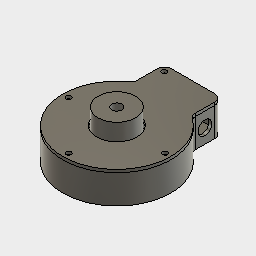
hihatController (Autodesk Fusion 360 design; units mm, degrees)
Autodesk Fusion 360 part; units mm, degrees
sketch "スケッチ1" plane through (0, 0, 0) normal (0, 1, 0) x (1, 0, 0)
  line L0 (-22, 22) -> (22, 22)
  line L1 (22, 22) -> (22, -22)
  line L2 (22, -22) -> (-22, -22)
  line L3 (-22, -22) -> (-22, 22)
  circle A0 centre (0, 0) radius 6.5
  circle A1 centre (0, 0) radius 37.5
  circle A2 centre (0, 0) radius 34.5
  line L4 (0, 47) -> (17.5, 47)
  line L5 (0, 47) -> (-17.5, 47)
  line L6 (-17.5, 47) -> (-17.5, 33.1662)
  line L7 (17.5, 47) -> (17.5, 33.1662)
  line L8 (-20.5, 33.1662) -> (-20.5, 31.4006)
  line L9 (20.5, 33.1662) -> (20.5, 31.4006)
  line L10 (-20.5, 31.4006) -> (-20.5, 25)
  line L11 (-17.5, 33.1662) -> (-17.5, 27)
  line L12 (17.5, 33.1662) -> (17.5, 26)
  line L13 (20.5, 31.4006) -> (20.5, 26)
  line L14 (-20.5, 50) -> (-20.5, 33.1662)
  line L15 (0, 50) -> (-20.5, 50)
  line L16 (0, 50) -> (20.5, 50)
  line L17 (20.5, 50) -> (20.5, 33.1662)
  dimension "d18" = 3
extrude "押し出し1" add sketch "スケッチ1" along normal blind 40 contours A1 A2 L10 L13 | A1 A2 L12 L13 | A1 L4 L5 L6 L7 L8 L9 L14 L15 L16 L17 | A1 A2 L10 L11 makes body 1
extrude "押し出し2" add sketch "スケッチ1" along normal blind 3 contours L0 L1 L2 L3 | A1 A2 L11 L12 | A1 L4 L5 L6 L7 | A2 bodies 1
fillet "フィレット1" radius 10 2 edges at (20.5, 20, -31.4006) (-20.5, 20, -31.4006) on bodies 1
fillet "フィレット2" radius 5 2 edges at (-20.5, 20, -50) (20.5, 20, -50) on bodies 1
fillet "フィレット3" radius 2 2 edges at (-17.5, 21.5, -47) (17.5, 21.5, -47) on bodies 1
sketch "スケッチ2" plane through (20.5, 0, 0) normal (1, 0, 0) x (0, 0, -1)
  line L0 (45, 0) -> (45, 40)
  line L1 (45, 40) -> (36.4143, 40)
  line L2 (36.4143, 40) -> (36.4143, 0)
  line L3 (36.4143, 0) -> (45, 0)
  line L4 (40.7071, 0) -> (40.7071, 10)
  circle A0 centre (40.7071, 10) radius 4.75
  dimension "d26" = 10
  dimension "d27" = 9.5
  measures "d26" distance of L4.start L4.end
  measures "d27" diameter of A0
extrude "押し出し3" cut sketch "スケッチ2" along normal mid plane 14 contours L0 L2 A0 | L0 A0 | L2 A0 bodies 1
sketch "スケッチ3" plane through (0, 40, 0) normal (0, 1, 0) x (-1, 0, 0)
  arc A0 (-20.5, -45) -> (-15.5, -50) centre (-15.5, -45) ccw
  line L0 (-15.5, -50) -> (15.5, -50)
  arc A1 (15.5, -50) -> (20.5, -45) centre (15.5, -45) ccw
  line L1 (20.5, -45) -> (20.5, -36.4143)
  arc A2 (24.0789, -28.7481) -> (20.5, -36.4143) centre (30.5, -36.4143) ccw
  arc A3 (24.0789, -28.7481) -> (-24.0789, -28.7481) centre (0, 0) ccw
  arc A4 (-20.5, -36.4143) -> (-24.0789, -28.7481) centre (-30.5, -36.4143) ccw
  line L2 (-20.5, -36.4143) -> (-20.5, -45)
  line L3 (15.5, -47) -> (-15.5, -47)
  arc A5 (-17.5, -45) -> (-15.5, -47) centre (-15.5, -45) ccw
  line L4 (-17.5, -45) -> (-17.5, -29.7321)
  arc A6 (17.5, -29.7321) -> (-17.5, -29.7321) centre (0, 0) ccw
  line L5 (17.5, -29.7321) -> (17.5, -45)
  arc A7 (15.5, -47) -> (17.5, -45) centre (15.5, -45) ccw
  circle A8 centre (0, 0) radius 37.5
  circle A9 centre (0, 0) radius 37.5
  circle A10 centre (0, 0) radius 34.5
  circle A11 centre (0, 0) radius 34.5
  circle A12 centre (0, 0) radius 56.7387
  point P0 (-10.5, -40)
  point P1 (10.5, -40)
extrude "押し出し4" cut sketch "スケッチ3" against normal blind 20 contours A0 L0 A1 L1 A2 A4 L2 L3 A5 L4 L5 A7 A8 A9 | L3 A5 L4 L5 A7 A8 A9 | A12 bodies 1
extrude "押し出し5" add sketch "スケッチ3" against normal blind 20 contours L4 L5 A8 A9 A10 A11 bodies 1
sketch "スケッチ4" plane through (0, 20, 0) normal (0, 1, 0) x (-1, 0, 0)
  line L0 (17.5, -33.1662) -> (17.5, -45)
  arc A0 (15.5, -47) -> (17.5, -45) centre (15.5, -45) ccw
  line L1 (15.5, -47) -> (-15.5, -47)
  arc A1 (-17.5, -45) -> (-15.5, -47) centre (-15.5, -45) ccw
  line L2 (-17.5, -45) -> (-17.5, -33.1662)
  arc A2 (-24.0789, -28.7481) -> (-17.5, -33.1662) centre (0, 0) ccw
  arc A3 (-20.5, -36.4143) -> (-24.0789, -28.7481) centre (-30.5, -36.4143) ccw
  line L3 (-20.5, -36.4143) -> (-20.5, -45)
  arc A4 (-20.5, -45) -> (-15.5, -50) centre (-15.5, -45) ccw
  line L4 (-15.5, -50) -> (15.5, -50)
  arc A5 (15.5, -50) -> (20.5, -45) centre (15.5, -45) ccw
  line L5 (20.5, -45) -> (20.5, -36.4143)
  arc A6 (24.0789, -28.7481) -> (20.5, -36.4143) centre (30.5, -36.4143) ccw
  arc A7 (17.5, -33.1662) -> (24.0789, -28.7481) centre (0, 0) ccw
  circle A8 centre (0, 0) radius 37.5
  arc A9 (-17.5, -33.1662) -> (17.5, -33.1662) centre (0, 0) ccw
  circle A10 centre (0, 0) radius 37.5
  point P0 (-15.5, -45)
  point P1 (15.5, -45)
sketch "スケッチ5" plane through (20.5, 0, 0) normal (1, 0, 0) x (0, 0, -1)
  line L0 (36.4143, 20) -> (36.4143, 12.0332)
  arc A0 (45, 12.0332) -> (36.4143, 12.0332) centre (40.7071, 10) ccw
  line L1 (45, 12.0332) -> (45, 20)
  arc A1 (36.4143, 7.9668) -> (45, 7.9668) centre (40.7071, 10) ccw
  line L2 (40.7071, 14.75) -> (40.7071, 5.25)
  circle A2 centre (40.7071, 10) radius 7.5
  circle A3 centre (40.7071, 10) radius 4.75
  line L3 (36.4143, 0) -> (36.4143, 16.1499)
  line L4 (45, 20) -> (36.4143, 20)
  point P0 (36.4143, 0)
  dimension "d37" = 15
  measures "d37" diameter of A2
extrude "押し出し7" add sketch "スケッチ5" against normal blind 1 contours L0 A0 L1 A2 A3 L3 | L0 A2 A3 L3 | L1 A1 A2 A3 L3 bodies 1
extrude "押し出し8" cut sketch "スケッチ5" along normal blind 2 contours L0 A2 A3 L3 bodies 1
sketch "スケッチ6" plane through (30.5, 0, 0) normal (1, 0, 0) x (0, 0, -1)
  circle A0 centre (40.7071, 10) radius 4.75
  circle A1 centre (40.7071, 10) radius 6
  line L0 (34.7071, 10) -> (34.7071, 1)
  line L1 (34.7071, 1) -> (45.4811, 1)
  line L2 (34.7071, 10) -> (46.7068, 10)
  line L3 (46.7068, 10) -> (46.7068, 1)
  line L4 (46.7068, 1) -> (45.4811, 1)
  point P0 (34.7071, 10)
  dimension "d45" = 11.9996
  measures "d45" distance of P0 L2.end
sketch "スケッチ7" plane through (19.5, 0, 0) normal (-1, 0, 0) x (0, 0, 1)
  line L0 (-48, 8.2495) -> (-48, 11.7505)
  arc A0 (-48, 11.7505) -> (-48, 8.2495) centre (-40.7071, 10) ccw
extrude "押し出し11" add sketch "スケッチ7" along normal blind 1 bodies 1
extrude "押し出し12" add sketch "スケッチ4" along normal mid plane 2 contours L0 A0 L1 A1 L2 A2 A3 L3 A4 L4 A5 L5 A6 A7 A8 A10 | L0 A0 L1 A1 L2 A8 A9 A10 bodies 1
extrude "押し出し13" add sketch "スケッチ5" along normal blind 1 contours L0 A0 L1 A2 A3 L3 | L0 A2 A3 L3 | L1 A1 A2 A3 L3 bodies 1
sketch "スケッチ8" plane through (0, 0, 0) normal (0, 1, 0) x (1, 0, 0)
  circle A0 centre (0, 0) radius 6.5
  circle A1 centre (0, 0) radius 6.5
  circle A2 centre (0, 0) radius 37.5
  arc A3 (-24.0789, 28.7481) -> (24.0789, 28.7481) centre (0, 0) ccw
  circle A4 centre (0, 0) radius 34.5
  arc A5 (-17.5, 29.7321) -> (17.5, 29.7321) centre (0, 0) ccw
  arc A6 (17.5, 33.1662) -> (-17.5, 33.1662) centre (0, 0) ccw
  line L0 (-15.5, 50) -> (15.5, 50)
  line L1 (0, 37.5) -> (0, 53)
  line L2 (0, 53) -> (20, 53)
  line L3 (20, 53) -> (-20, 53)
  line L4 (-20, 53) -> (-20, 26)
  line L5 (20, 53) -> (20, 23)
  line L6 (-18, 51) -> (-18, 26)
  line L7 (18, 51) -> (-18, 51)
  line L8 (18, 51) -> (18, 23)
  dimension "d62" = 40
  dimension "d63" = 2
  measures "d62" distance of L2.end L3.end
extrude "押し出し14" add sketch "スケッチ8" along normal blind 20 separate body contours A2 A3 A4 A5 L4 L5 | A2 A4 A5 L5 L8 | A2 A4 A5 L4 L6 | A2 A4 A5 A6 L6 L8 makes body 2
extrude "押し出し15" add sketch "スケッチ8" along normal blind 3 contours A4 A5 bodies 2
extrude "押し出し16" cut sketch "スケッチ8" along normal blind 20 contours A2 A4 A5 A6 L6 L8 bodies 2
extrude "押し出し17" add sketch "スケッチ8" along normal blind 20 contours A2 L1 L2 L3 L5 L7 L8 | A2 L1 L3 L4 L6 L7 bodies 2
extrude "押し出し18" add sketch "スケッチ8" along normal blind 3 contours A2 A4 A5 A6 L6 L8 | A2 A6 L1 L7 L8 | A2 A6 L1 L6 L7 bodies 2
fillet "フィレット8" radius 5 2 edges at (-20, 10, -31.7214) (20, 10, -31.7214) on bodies 2
fillet "フィレット9" radius 5 2 edges at (-20, 10, -53) (20, 10, -53) on bodies 2
fillet "フィレット10" radius 4 2 edges at (18, 11.5, -51) (-18, 11.5, -51) on bodies 2
sketch "スケッチ9" plane through (20, 0, 0) normal (1, 0, 0) x (0, 0, -1)
  line L0 (48, 0) -> (48, 20)
  line L1 (48, 20) -> (34.3693, 20)
  line L2 (34.3693, 20) -> (34.3693, 0)
  line L3 (34.3693, 0) -> (48, 0)
  line L4 (41.1847, 0) -> (41.1847, 10)
  circle A0 centre (41.1847, 10) radius 4.75
  dimension "d73" = 9.5
  measures "d73" diameter of A0
extrude "押し出し19" cut sketch "スケッチ9" against normal blind 2 contours A0 bodies 2
sketch "スケッチ10" plane through (0, 20, 0) normal (0, 1, 0) x (-1, 0, 0)
  arc A0 (-20, -48) -> (-15, -53) centre (-15, -48) ccw
  line L0 (-15, -53) -> (15, -53)
  arc A1 (15, -53) -> (20, -48) centre (15, -48) ccw
  line L1 (20, -48) -> (20, -34.3693)
  arc A2 (22.0588, -30.3259) -> (20, -34.3693) centre (25, -34.3693) ccw
  arc A3 (22.0588, -30.3259) -> (-22.0588, -30.3259) centre (0, 0) ccw
  arc A4 (-20, -34.3693) -> (-22.0588, -30.3259) centre (-25, -34.3693) ccw
  line L2 (-20, -34.3693) -> (-20, -48)
  line L3 (18, -29.4321) -> (18, -47)
  arc A5 (14, -51) -> (18, -47) centre (14, -47) ccw
  line L4 (14, -51) -> (-14, -51)
  arc A6 (-18, -47) -> (-14, -51) centre (-14, -47) ccw
  line L5 (-18, -47) -> (-18, -29.4321)
  arc A7 (18, -29.4321) -> (-18, -29.4321) centre (0, 0) ccw
  circle A8 centre (0, 0) radius 34.5
sketch "スケッチ11" plane through (0, 20, 0) normal (0, 1, 0) x (-1, 0, 0)
  arc A0 (-20, -48) -> (-15, -53) centre (-15, -48) ccw
  line L0 (-15, -53) -> (15, -53)
  arc A1 (15, -53) -> (20, -48) centre (15, -48) ccw
  line L1 (20, -48) -> (20, -34.3693)
  arc A2 (22.0588, -30.3259) -> (20, -34.3693) centre (25, -34.3693) ccw
  arc A3 (22.0588, -30.3259) -> (-22.0588, -30.3259) centre (0, 0) ccw
  arc A4 (-20, -34.3693) -> (-22.0588, -30.3259) centre (-25, -34.3693) ccw
  line L2 (-20, -34.3693) -> (-20, -48)
  circle A5 centre (0, 0) radius 30
  line L3 (18, -29.4321) -> (18, -47)
  arc A6 (14, -51) -> (18, -47) centre (14, -47) ccw
  line L4 (14, -51) -> (-14, -51)
  arc A7 (-18, -47) -> (-14, -51) centre (-14, -47) ccw
  line L5 (-18, -47) -> (-18, -29.4321)
  arc A8 (18, -29.4321) -> (-18, -29.4321) centre (0, 0) ccw
  dimension "d78" = 60
  measures "d78" diameter of A5
extrude "押し出し21" add sketch "スケッチ11" along normal blind 3 separate body contours A5 makes body 3
sketch "スケッチ12" plane through (0, 23, 0) normal (0, 1, 0) x (-1, 0, 0)
  circle A0 centre (0, 0) radius 30
  circle A1 centre (0, 0) radius 13
  dimension "d81" = 26
  measures "d81" diameter of A1
extrude "押し出し22" add sketch "スケッチ12" along normal blind 27 contours A1 bodies 3
sketch "スケッチ13" plane through (0, 50, 0) normal (0, 1, 0) x (-1, 0, 0)
  circle A0 centre (0, 0) radius 13
  circle A1 centre (0, 0) radius 3.25
  dimension "d84" = 6.5
  measures "d84" diameter of A1
extrude "押し出し23" cut sketch "スケッチ13" against normal blind 34 contours A1 bodies 3
sketch "スケッチ14" plane through (0, 3, 0) normal (0, 1, 0) x (-1, 0, 0)
  arc A0 (14, -51) -> (18, -47) centre (14, -47) ccw
  line L0 (18, -47) -> (18, -29.4321)
  arc A1 (18, -29.4321) -> (-18, -29.4321) centre (0, 0) ccw
  line L1 (-18, -29.4321) -> (-18, -47)
  arc A2 (-18, -47) -> (-14, -51) centre (-14, -47) ccw
  line L2 (-14, -51) -> (14, -51)
  circle A3 centre (0, 0) radius 6.5
  arc A4 (15, -53) -> (20, -48) centre (15, -48) ccw
  line L3 (18.5355, -51.5355) -> (13, -46)
  circle A5 centre (15.7678, -48.7678) radius 1.5
  circle A6 centre (15.7678, -48.7678) radius 3.9142
  arc A7 (22.0588, -30.3259) -> (-22.0588, -30.3259) centre (0, 0) ccw
  line L4 (-37.5, 0) -> (37.5, 0)
  line L5 (0, 37.5) -> (0, 0)
  line L6 (-34.5, 0) -> (-33.5, 0)
  circle A8 centre (-33.5, 0) radius 1.5
  circle A9 centre (-33.5, 0) radius 3
  line L7 (0, 34.5) -> (0, 33.5)
  circle A10 centre (0, 33.5) radius 1.5
  circle A11 centre (0, 33.5) radius 3
  line L8 (34.5, 0) -> (33.5, 0)
  circle A12 centre (33.5, 0) radius 1.5
  circle A13 centre (33.5, 0) radius 3
  dimension "d87" = 3
  dimension "d88" = 1
  dimension "d89" = 3
  dimension "d90" = 1
  dimension "d91" = 3
  dimension "d92" = 6
  dimension "d93" = 1
  dimension "d94" = 3
  dimension "d95" = 6
  measures "d87" diameter of A5
  measures "d88" distance of L6.start L6.end
  measures "d89" diameter of A8
  measures "d90" distance of L7.start L7.end
  measures "d91" diameter of A10
  measures "d92" diameter of A11
  measures "d93" distance of L8.start L8.end
  measures "d94" diameter of A12
  measures "d95" diameter of A13
extrude "押し出し24" add sketch "スケッチ14" along normal blind 17 separate body contours A0 L2 L3 A5 A6 | A0 L0 L3 A5 A6 | A1 L4 A12 A13 | A1 L4 A8 A9 | A1 L4 A12 A13 | A1 L4 A8 A9 | A1 L5 A10 A11 | A1 L5 A10 A11 picked at (33.8892, -2.2584) picked at (-33.8892, -2.2584) picked at (33.8892, 2.2584) picked at (-33.8892, 2.2584) picked at (2.2535, 33.9782) picked at (-2.2584, 33.8892) makes body 4 at (34.0909, 14.3333, -2.9412) makes body 5 at (-33.6462, 8.6667, 2.9964) makes body 6 at (-11.9901, 14.3333, -49.7926) makes body 7 at (2.9964, 14.3333, 33.6462)
extrude "押し出し25" cut sketch "スケッチ14" along normal blind 25 contours A1 L4 A12 | A1 L4 A8 | A1 L4 A12 | A1 L4 A8 | A1 L5 A10 | A1 L5 A10 bodies 2
combine "結合1" operation add target body 2 tool bodies 5 7 4 6
move_body "移動3" bodies 3 to x (1, 0, 0) y (0, 1, 0) z (0, 0, 1) at (0, -7, 0)
sketch "スケッチ15" plane through (0, 16, 0) normal (0, 1, 0) x (-1, 0, 0)
  circle A0 centre (0, 0) radius 13
  circle A1 centre (0, 0) radius 30
  line L0 (30, 0) -> (29.5, 0)
  circle A2 centre (0, 0) radius 29.5
  dimension "d100" = 0.5
  measures "d100" distance of L0.start L0.end
extrude "押し出し26" cut sketch "スケッチ15" against normal blind 3 contours A1 bodies 3
sketch "スケッチ16" plane through (0, 16, 0) normal (0, 1, 0) x (-1, 0, 0)
  circle A0 centre (0, 0) radius 29.5
  circle A1 centre (0, 0) radius 13
  line L0 (0, 0) -> (-29.5, 0)
  arc A2 (34.3806, 2.8678) -> (34.3806, -2.8678) centre (33.5, 0) ccw
  line L1 (0, 0) -> (30.5, 0)
  line L2 (0, 0) -> (0, -32)
  line L3 (0, 0) -> (0, 30)
  line L4 (5, -5) -> (5, -32)
  line L5 (5, -5) -> (30.5, -5)
  line L6 (-5, 5) -> (-5, 30)
  line L7 (-5, 5) -> (-29.5, 5)
  line L8 (-5, -5) -> (-5, -32)
  line L9 (-5, -5) -> (-29.5, -5)
  line L10 (5, 5) -> (5, 30)
  line L11 (5, 5) -> (30.5, 5)
  point P0 (-29.5, 0)
  dimension "d103" = 5
  dimension "d104" = 5
  dimension "d105" = 5
  dimension "d106" = 5
extrude "押し出し27" add sketch "スケッチ16" along normal blind 3.5 contours A0 A1 L1 L11 | A0 A1 L1 L5 | A0 A1 L3 L10 | A0 A1 L2 L4 | A0 A1 L3 L6 | A0 A1 L2 L8 | A0 A1 L0 L7 | A0 A1 L0 L9 bodies 3
sketch "スケッチ17" plane through (0, 20, 0) normal (0, 1, 0) x (-1, 0, 0)
  circle A0 centre (15.7678, -48.7678) radius 1.5
  arc A1 (18, -45.5525) -> (12.5525, -51) centre (15.7678, -48.7678) ccw
  line L0 (12.5525, -51) -> (-14, -51)
  arc A2 (-18, -47) -> (-14, -51) centre (-14, -47) ccw
  line L1 (-18, -47) -> (-18, -29.4321)
  arc A3 (-34.3806, -2.8678) -> (-18, -29.4321) centre (0, 0) ccw
  arc A4 (-34.3806, -2.8678) -> (-34.3806, 2.8678) centre (-33.5, 0) ccw
  arc A5 (-2.8678, 34.3806) -> (-34.3806, 2.8678) centre (0, 0) ccw
  arc A6 (-2.8678, 34.3806) -> (2.8678, 34.3806) centre (0, 33.5) ccw
  arc A7 (34.3806, 2.8678) -> (2.8678, 34.3806) centre (0, 0) ccw
  arc A8 (34.3806, 2.8678) -> (34.3806, -2.8678) centre (33.5, 0) ccw
  arc A9 (18, -29.4321) -> (34.3806, -2.8678) centre (0, 0) ccw
  line L2 (18, -29.4321) -> (18, -45.5525)
  circle A10 centre (-33.5, 0) radius 1.5
  circle A11 centre (0, 33.5) radius 1.5
  circle A12 centre (33.5, 0) radius 1.5
  arc A13 (-20, -48) -> (-15, -53) centre (-15, -48) ccw
  line L3 (-15, -53) -> (15, -53)
  arc A14 (15, -53) -> (20, -48) centre (15, -48) ccw
  line L4 (20, -48) -> (20, -34.3693)
  arc A15 (22.0588, -30.3259) -> (20, -34.3693) centre (25, -34.3693) ccw
  arc A16 (22.0588, -30.3259) -> (-22.0588, -30.3259) centre (0, 0) ccw
  arc A17 (-20, -34.3693) -> (-22.0588, -30.3259) centre (-25, -34.3693) ccw
  line L5 (-20, -34.3693) -> (-20, -48)
  circle A18 centre (0, 0) radius 14
  dimension "d109" = 28
  measures "d109" diameter of A18
extrude "押し出し28" add sketch "スケッチ17" along normal blind 2 separate body contours A1 L0 A2 L1 A3 A4 A5 A6 A7 A8 A9 L2 | A13 L3 A14 L4 A15 A16 A17 L5 makes body 8
sketch "スケッチ18" plane through (0, 13, 0) normal (0, -1, 0) x (1, 0, 0)
  circle A0 centre (0, 0) radius 29.5
  circle A1 centre (0, 0) radius 3.25
  circle A2 centre (0, 0) radius 6.5
  dimension "d112" = 13
  measures "d112" diameter of A2
extrude "押し出し29" cut sketch "スケッチ18" against normal blind 15 contours A2 bodies 3
sketch "スケッチ19" plane through (0, 22, 0) normal (0, 1, 0) x (-1, 0, 0)
  circle A0 centre (-33.5, 0) radius 1.5
  circle A1 centre (33.5, 0) radius 1.5
  circle A2 centre (0, 0) radius 14
  circle A3 centre (15.7678, -48.7678) radius 1.5
  circle A4 centre (0, 33.5) radius 1.5
  arc A5 (22.0588, -30.3259) -> (-22.0588, -30.3259) centre (0, 0) ccw
  arc A6 (-20, -34.3693) -> (-22.0588, -30.3259) centre (-25, -34.3693) ccw
  line L0 (-20, -34.3693) -> (-20, -48)
  arc A7 (-20, -48) -> (-15, -53) centre (-15, -48) ccw
  line L1 (-15, -53) -> (15, -53)
  arc A8 (15, -53) -> (20, -48) centre (15, -48) ccw
  line L2 (20, -48) -> (20, -34.3693)
  arc A9 (22.0588, -30.3259) -> (20, -34.3693) centre (25, -34.3693) ccw
  circle A10 centre (33.5, 0) radius 1.75
  circle A11 centre (15.7678, -48.7678) radius 1.75
  circle A12 centre (-33.5, 0) radius 1.75
  circle A13 centre (0, 33.5) radius 1.75
  circle A14 centre (0, 0) radius 34.5
  arc A15 (-34.3806, -2.8678) -> (-18, -29.4321) centre (0, 0) ccw
  line L3 (0, 0) -> (-20.5068, -27.7439)
  line L4 (-20.5068, -27.7439) -> (-19.9124, -26.9397)
  circle A16 centre (-19.9124, -26.9397) radius 1.5
  circle A17 centre (-19.9124, -26.9397) radius 3
  circle A18 centre (-19.9124, -26.9397) radius 1.75
  dimension "d115" = 3.5
  dimension "d116" = 3.5
  dimension "d117" = 3.5
  dimension "d118" = 3.5
  dimension "d119" = 1
  dimension "d120" = 3
  dimension "d121" = 6
  dimension "d122" = 3.5
  measures "d115" diameter of A10
  measures "d116" diameter of A11
  measures "d117" diameter of A12
  measures "d118" diameter of A13
  measures "d119" distance of L3.end L4.end
  measures "d120" diameter of A16
  measures "d121" diameter of A17
  measures "d122" diameter of A18
extrude "押し出し30" cut sketch "スケッチ19" against normal blind 2 contours A0 A12 A14 | A0 A12 A14 | A4 A13 A14 | A4 A13 A14 | A1 A10 A14 | A1 A10 A14 | A11 bodies 8
copy_body "ボディのコピーと貼り付け1" bodies 8 makes body 9
sketch "スケッチ20" plane through (0, 43, 0) normal (0, 1, 0) x (-1, 0, 0)
  circle A0 centre (0, 0) radius 3.25
  circle A1 centre (0, 0) radius 13
  circle A2 centre (0, 0) radius 3.5
  dimension "d125" = 7
  measures "d125" diameter of A2
extrude "押し出し31" cut sketch "スケッチ20" against normal blind 83 contours A2 bodies 3
copy_body "ボディのコピーと貼り付け2" bodies 3 makes body 10
move_face "面をオフセット3" offset -10 1 faces at (-9.7719, 43, -0.8197) on bodies 10
hidden bodies 1 3 9
named bodies: "rid", "rid2"
